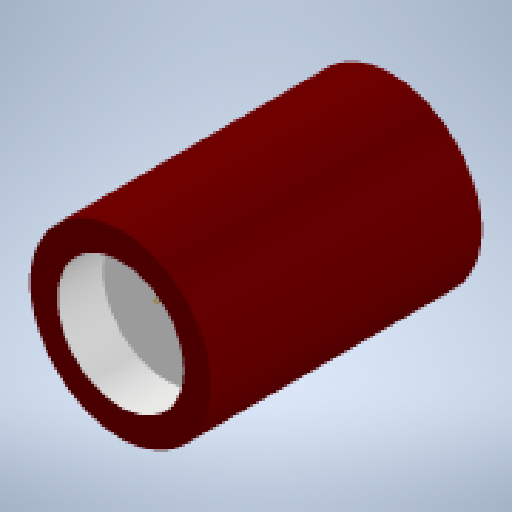
# Autodesk Inventor part: terminal
Saved by Autodesk Inventor 2024 (Build 280153000, 153)
## iProperties
Created: 2024-02-15
Part Number: terminal
Material: Generic
Document SubType Name: Modeling
Designer: fabiancastano
Density: 1 g/cm^3
Appearance: Default
Author: fabiancastano
Autodesk Inventor part; units mm, degrees
ref_plane "YZ Plane" through (0, 0, 0) normal (1, 0, 0) x (0, 1, 0)
ref_plane "XZ Plane" through (0, 0, 0) normal (0, 1, 0) x (-1, 0, 0)
ref_plane "XY Plane" through (0, 0, 0) normal (0, 0, 1) x (1, 0, 0)
sketch "Sketch1" plane through (0, 0, 0) normal (0, 0, 1) x (1, 0, 0)
  circle A0 centre (9.6513, 12.486) radius 1.25 projected
  circle A1 centre (9.6513, 12.486) radius 0.5
  point P0 (0, 0)
  dimension "d0" = 1
  constraints: 1 centre point, 1 coincident
  measures "d0" diameter of A1
extrude "Extrusion1" add sketch "Sketch1" along normal blind 1.5 contours A1
sketch "Sketch2" plane through (9.6513, 12.486, 1.5) normal (0, 0, 1) x (1, 0, 0)
  circle A0 centre (0, 0) radius 0.35
  point P0 (-9.6513, -12.486)
  dimension "d3" = 0.7
  constraints: 1 centre point
  measures "d3" diameter of A0
extrude "Extrusion2" cut sketch "Sketch2" against normal blind 0.254
sketch "Sketch3" plane through (9.6513, 12.486, 0) normal (0, 0, -1) x (-1, 0, 0)
  circle A0 centre (0, 0) radius 0.35
  point P0 (9.6513, -12.486)
  dimension "d6" = 0.7
  constraints: 1 centre point
  measures "d6" diameter of A0
extrude "Extrusion3" cut sketch "Sketch3" against normal blind 0.254
sketch "Sketch4" plane through (9.6513, 12.486, 0.254) normal (0, 0, -1) x (-1, 0, 0)
  circle A0 centre (0, 0) radius 0.35 projected
body "Solid1"
